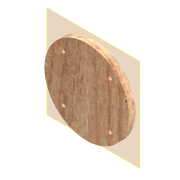
# Autodesk Inventor part: spacer lidar
Saved by Autodesk Inventor 2020.3 (Build 243373000, 373)
## iProperties
Created: 2020-12-10
Part Number: spacer lidar
Material: Wood (Birch)
Document SubType Name: Sheet Metal
Designer: Svend
Density: 0.55 g/cm^3
Sheet Metal Rule: Default_mm
Appearance: Birch - Natural Polished
Author: Svend
Autodesk Inventor part; units mm, degrees
ref_plane "YZ Plane" through (0, 0, 0) normal (1, 0, 0) x (0, 1, 0)
ref_plane "XZ Plane" through (0, 0, 0) normal (0, 1, 0) x (-1, 0, 0)
ref_plane "XY Plane" through (0, 0, 0) normal (0, 0, 1) x (1, 0, 0)
ref_plane "Work Plane1" through (0, 0, 0) normal (0, 0, 1) x (1, 0, 0)
sketch "Sketch1" plane through (0, 0, 0) normal (0, 0, 1) x (1, 0, 0)
  circle A0 centre (-20.75, 20.75) radius 1.5
  circle A1 centre (-20.75, -20.75) radius 1.5
  circle A2 centre (20.75, 20.75) radius 1.5
  circle A3 centre (20.75, -20.75) radius 1.5
  circle A4 centre (0, 0) radius 37.5402
extrude "Plate1" add sketch "Sketch1" along normal blind 6
equation "\"d0\" = Thickness"
equation "\"BendRadius\" = Thickness"
equation "\"BendReliefWidth\" = Thickness"
equation "\"BendReliefDepth\" = 0.5 * Thickness"
equation "\"CornerReliefSize\" = 4 * Thickness"
equation "\"MinimumRemnant\" = 2 * Thickness"
equation "\"TransitionRadius\" = BendRadius"
equation "\"JacobiRadiusSize\" = BendRadius"
equation "\"GapSize\" = Thickness"
equation "\"Thickness\" = 6"
body "Solid1"
